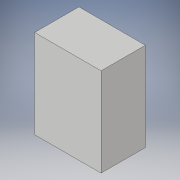
# Autodesk Inventor part: Electrical Box Placeholder
Saved by Autodesk Inventor 2019 (Build 230136000, 136)
## iProperties
Created: 2018-10-28
Part Number: Electrical Box Placeholder
Material: Generic
Document SubType Name: Modeling
Designer: Swapnil
Density: 1 g/cm^3
Appearance: Default
Author: Swapnil
Autodesk Inventor part; units mm, degrees
ref_plane "YZ Plane" through (0, 0, 0) normal (1, 0, 0) x (0, 1, 0)
ref_plane "XZ Plane" through (0, 0, 0) normal (0, 1, 0) x (-1, 0, 0)
ref_plane "XY Plane" through (0, 0, 0) normal (0, 0, 1) x (1, 0, 0)
sketch "Sketch1" plane through (0, 0, 0) normal (0, 0, 1) x (1, 0, 0)
  line L0 (0, 0) -> (0, 168.7484) construction
  line L1 (0, 0) -> (186.2051, 0) construction
  line L2 (-76.2, 101.6) -> (76.2, 101.6)
  line L3 (76.2, 101.6) -> (76.2, -101.6)
  line L4 (76.2, -101.6) -> (-76.2, -101.6)
  line L5 (-76.2, -101.6) -> (-76.2, 101.6)
  dimension "d0" = 203.2
  dimension "d1" = 152.4
  constraints: 12 end point, 2 horizontal, 2 parallel, 1 perpendicular, 1 vertical, 2 other
  measures "d0" distance of L2.end L3.end
  measures "d1" distance of L2.start L2.end
extrude "Extrusion1" add sketch "Sketch1" along normal blind 101.6
body "Solid1"
